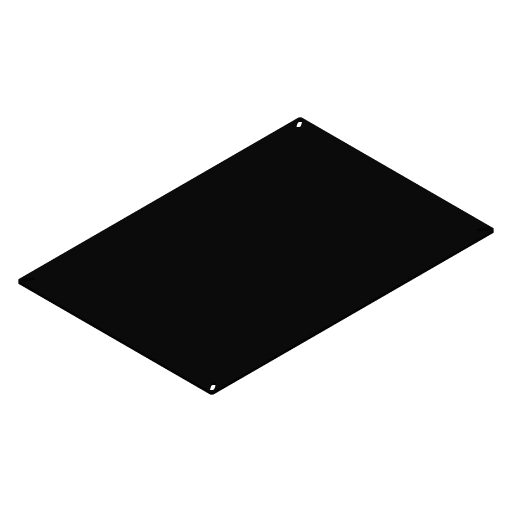
# Autodesk Inventor part: E3D High Temperature Bed 300x200
Saved by Autodesk Inventor 2023.2 (Build 272271000, 271)
## iProperties
Created: 2023-02-02
Part Number: E3D High Temperature Bed 300x200
Material: Copper
Document SubType Name: Modeling
Designer: remop
Density: 8.94 g/cm^3
Appearance: Anodized - Black
Author: remop
Autodesk Inventor part; units mm, degrees
ref_plane "YZ Plane" through (0, 0, 0) normal (1, 0, 0) x (0, 1, 0)
ref_plane "XZ Plane" through (0, 0, 0) normal (0, 1, 0) x (-1, 0, 0)
ref_plane "XY Plane" through (0, 0, 0) normal (0, 0, 1) x (1, 0, 0)
sketch "Sketch1" plane through (0, 0, 0) normal (0, 1, 0) x (-1, 0, 0)
  line L0 (-108, -157) -> (108, -157)
  line L1 (108, -157) -> (108, 157)
  line L2 (108, 157) -> (-108, 157)
  line L3 (-108, 157) -> (-108, -157)
  line L4 (-108, -157) -> (108, 157) construction
  line L5 (108, -157) -> (-108, 157) construction
  line L6 (104.5, 153.5) -> (100.3061, 147.2822) construction
  line L7 (102.8419, 154.6184) -> (98.648, 148.4006)
  line L8 (101.9641, 146.1638) -> (106.1581, 152.3816)
  arc A0 (106.1581, 152.3816) -> (102.8419, 154.6184) centre (104.5, 153.5) ccw
  arc A1 (98.648, 148.4006) -> (101.9641, 146.1638) centre (100.3061, 147.2822) ccw
  line L9 (0, -219.8) -> (0, 219.8) projected
  line L10 (151.2, 0) -> (-151.2, 0) projected
  line L11 (-102.8419, 154.6184) -> (-98.648, 148.4006)
  line L12 (-101.9641, 146.1638) -> (-106.1581, 152.3816)
  arc A2 (-102.8419, 154.6184) -> (-106.1581, 152.3816) centre (-104.5, 153.5) ccw
  arc A3 (-101.9641, 146.1638) -> (-98.648, 148.4006) centre (-100.3061, 147.2822) ccw
  line L13 (102.8419, -154.6184) -> (98.648, -148.4006)
  line L14 (101.9641, -146.1638) -> (106.1581, -152.3816)
  arc A4 (102.8419, -154.6184) -> (106.1581, -152.3816) centre (104.5, -153.5) ccw
  arc A5 (101.9641, -146.1638) -> (98.648, -148.4006) centre (100.3061, -147.2822) ccw
  line L15 (-101.9641, -146.1638) -> (-106.1581, -152.3816)
  arc A6 (-106.1581, -152.3816) -> (-102.8419, -154.6184) centre (-104.5, -153.5) ccw
  line L16 (-102.8419, -154.6184) -> (-98.648, -148.4006)
  arc A7 (-98.648, -148.4006) -> (-101.9641, -146.1638) centre (-100.3061, -147.2822) ccw
  point P0 (0, 0)
  point P1 (102.403, 150.3911)
  dimension "d0" = 314
  dimension "d1" = 216
  dimension "d2" = 7.5
  dimension "d3" = 3.5
  dimension "d4" = 3.5
  dimension "d5" = 2
  dimension "d6" = 34
  constraints: 32 end point, 18 symmetric about line, 16 point on circle, 8 centre point, 4 tangent, 3 midpoint, 3 parallel, 1 horizontal, 1 perpendicular, 6 other
  measures "d0" distance of L0.end L1.end
  measures "d1" distance of L1.end L2.end
  measures "d2" distance of L6.start L6.end
  measures "d3" distance from line of L1 L6.start
  measures "d4" distance from line of L2 L6.start
  measures "d5" radius of A1
  measures "d6" angle of L1 L8
extrude "Extrusion1" add sketch "Sketch1" along normal blind 3
fillet "Fillet1" radius 2 4 edges at (108, 1.5, 157) (108, 1.5, -157) (-108, 1.5, -157) (-108, 1.5, 157)
body "Solid1"
